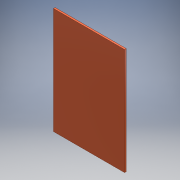
# Autodesk Inventor part: Antenna
Saved by Autodesk Inventor 2017 (Build 210142000, 142)
## iProperties
Created: 2018-07-07
Part Number: Antenna
Material: Copper, Wrought
Document SubType Name: Modeling
Designer: Galindo
Density: 8.94 g/cm^3
Appearance: Copper - Satin
Author: Galindo
Autodesk Inventor part; units mm, degrees
ref_plane "YZ Plane" through (0, 0, 0) normal (1, 0, 0) x (0, 1, 0)
ref_plane "XZ Plane" through (0, 0, 0) normal (0, 1, 0) x (-1, 0, 0)
ref_plane "XY Plane" through (0, 0, 0) normal (0, 0, 1) x (1, 0, 0)
sketch "Sketch1" plane through (0, 0, 0) normal (0, 1, 0) x (-1, 0, 0)
  line L0 (0, 0) -> (-10, 0)
  line L1 (-10, 0) -> (-10, -15)
  line L2 (-10, -15) -> (0, -15)
  line L3 (0, -15) -> (0, 0)
  dimension "d0" = 15
  dimension "d1" = 10
  constraints: 8 end point, 2 parallel, 1 horizontal, 1 perpendicular
  measures "d0" distance of L0.end L1.end
  measures "d1" distance of L1.end L2.end
extrude "Extrusion1" add sketch "Sketch1" along normal blind 0.23
sketch "Sketch2" plane through (0, 0.23, 0) normal (0, 1, 0) x (1, 0, 0)
  line L0 (4.68, 10.01) -> (3.2, 10.01)
  line L1 (3.2, 10.01) -> (3.2, 11.99)
  line L2 (3.2, 11.99) -> (4.68, 11.99)
  line L3 (4.68, 11.99) -> (4.68, 10.01)
  line L4 (1.48, 10.01) -> (0, 10.01)
  line L5 (0, 10.01) -> (0, 11.99)
  line L6 (0, 11.99) -> (1.48, 11.99)
  line L7 (1.48, 11.99) -> (1.48, 10.01)
  line L8 (0, 11.99) -> (1.48, 10.01) construction
  line L9 (3.2, 11.99) -> (4.68, 10.01) construction
  line L10 (10, 15) -> (0, 15) construction
  line L11 (10, 0) -> (10, 15) construction
  line L12 (0, 15) -> (0, 0) projected
  point P0 (0.74, 11)
  point P1 (3.94, 11)
  dimension "d4" = 3.2
  dimension "d5" = 4
  dimension "d6" = 1.48
  dimension "d7" = 1.98
  constraints: 20 end point, 5 parallel, 4 collinear, 2 horizontal, 2 midpoint, 2 perpendicular
  measures "d4" distance of point (3.94, 11) point (0.74, 11)
  measures "d5" distance from line of point (3.94, 11) L10
  measures "d6" distance of L0.start L0.end
  measures "d7" distance of L4.end L5.end
extrude "Extrusion2" add sketch "Sketch2" along normal blind 0.035
body "Solid1"
